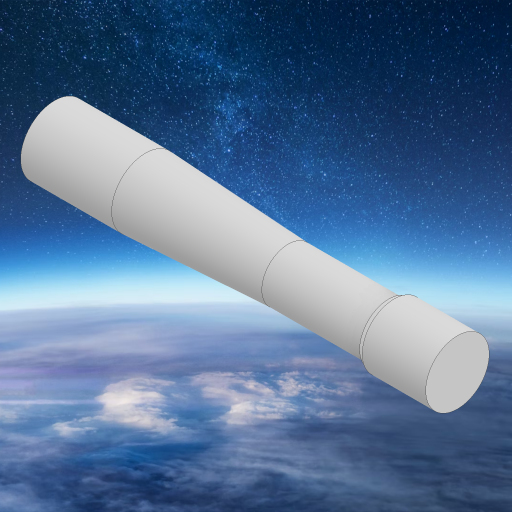
# Autodesk Inventor part: stick_antenna_434MHz
Saved by Autodesk Inventor 2023 (Build 270158000, 158)
## iProperties
Created: 2023-10-30
Part Number: stick_antenna_434MHz
Material: 一般
Document SubType Name: Modeling
Designer: 310611102
Density: 1 g/cm^3
Appearance: 預設
Author: 310611102
Autodesk Inventor part; units mm, degrees
ref_plane "YZ Plane" through (0, 0, 0) normal (1, 0, 0) x (0, 1, 0)
ref_plane "XZ Plane" through (0, 0, 0) normal (0, 1, 0) x (-1, 0, 0)
ref_plane "XY Plane" through (0, 0, 0) normal (0, 0, 1) x (1, 0, 0)
sketch "Sketch1" plane through (0, 0, 0) normal (0, 0, 1) x (1, 0, 0)
  line L0 (0, 0) -> (76.2, 0)
  line L1 (76.2, 0) -> (76.2, 6)
  line L2 (17.2, 6.4) -> (0, 6.4)
  line L3 (0, 6.4) -> (0, 3)
  line L4 (0, 0) -> (101.0496, 0)
  line L5 (76.2, 6) -> (64.2, 6)
  line L6 (64.2, 6) -> (63.2, 5.5)
  line L7 (63.2, 5.5) -> (63.2, 5)
  line L8 (63.2, 5) -> (44.2, 5)
  line L9 (44.2, 5) -> (17.2, 6.4)
  line L10 (0, 3) -> (5, 3)
  line L11 (5, 3) -> (5, 0)
  point P0 (5, 0)
  dimension "d0" = 76.2
  dimension "d1" = 12.8
  dimension "d3" = 12
  dimension "d4" = 10
  dimension "d5" = 0.5
  dimension "d6" = 1
  dimension "d7" = 13
  dimension "d8" = 32
  dimension "d9" = 59
  dimension "d10" = 5
  dimension "d11" = 6
  constraints: 24 end point, 4 horizontal, 3 perpendicular, 2 parallel, 2 point on line, 1 vertical
  measures "d0" distance of L0.start L0.end
  measures "d1" diameter of L2 L4
  measures "d3" diameter of L5 L4
  measures "d4" diameter of L8 L4
  measures "d5" distance of L6.end L7.end
  measures "d6" distance from line of L5.end L7
  measures "d7" distance between parallel lines of L1 L7
  measures "d8" distance from line of L1 L8.end
  measures "d9" distance from line of L2.start L1
  measures "d10" distance between parallel lines of L3 L11
  measures "d11" diameter of L10 L4
revolve "Revolution1" add sketch "Sketch1" angle 360 about axis through (0, 0, 0) along (1, 0, 0)
body "Solid1"
